Autodesk Inventor part; units mm, degrees
(part 2 of 2)
  spline S10 degree 5 poles (30.7335, -5.459) (30.6894, -5.4223) (30.6454, -5.3856) (30.6013, -5.349) (30.5128, -5.276) (30.4236, -5.2038) (30.3788, -5.168) (30.2889, -5.0968) (30.198, -5.0268) (30.1524, -4.992) (30.0608, -4.9229) (29.9686, -4.8547) (29.9224, -4.8208) (29.8295, -4.7535) (29.7359, -4.6872) (29.6889, -4.6543) (29.5946, -4.589) (29.4996, -4.5247) (29.4519, -4.4929) (29.3561, -4.4297) (29.2597, -4.3677) (29.2112, -4.3369) (29.114, -4.2761) (29.016, -4.2164) (28.9669, -4.1869) (28.8682, -4.1285) (28.7687, -4.0713) (28.7188, -4.0431) (28.6186, -3.9873) (28.5176, -3.9329) (28.4669, -3.906) (28.3651, -3.8531) (28.2626, -3.8017) (28.2111, -3.7764) (28.1077, -3.7267) (28.0035, -3.6787) (27.9512, -3.6551) (27.8462, -3.6092) (27.7402, -3.5651) (27.6871, -3.5436) (27.5804, -3.5014) (27.4729, -3.4613) (27.419, -3.4418) (27.3105, -3.4043) (27.201, -3.3704) (27.1459, -3.3543) (27.0348, -3.3257) (26.9231, -3.2995) (26.8672, -3.2864) (26.7557, -3.2591) (26.6453, -3.2277) (26.5905, -3.2106) (26.4821, -3.1729) (26.3763, -3.1281) (26.3244, -3.1036) (26.2219, -3.0515) (26.1238, -2.9918) (26.0756, -2.9603) (25.983, -2.8924) (25.8981, -2.8146) (25.8596, -2.7722) (25.7804, -2.6886) (25.7171, -2.5923) (25.6878, -2.5432) (25.6326, -2.442) (25.5979, -2.3325) (25.5767, -2.2787) (25.5598, -2.1649) (25.5445, -2.0515) (25.5485, -1.9934) (25.5547, -1.8796) (25.5649, -1.7651) (25.5676, -1.7081) (25.5752, -1.5936) (25.5834, -1.4798) (25.5913, -1.4224) (25.6225, -1.3127) (25.658, -1.2036) (25.6879, -1.1544) (25.737, -1.0509) (25.8098, -0.9618) (25.8435, -0.916) (25.9234, -0.8334) (26.0119, -0.7613) (26.0571, -0.7261) (26.1519, -0.6617) (26.2538, -0.6093) (26.3056, -0.5851) (26.411, -0.5405) (26.5196, -0.5041) (26.5744, -0.4877) (26.6851, -0.4586) (26.7974, -0.4368) (26.8539, -0.4278) (26.9673, -0.4125) (27.0811, -0.4011) (27.138, -0.3958) (27.2519, -0.385) (27.3654, -0.3711) (27.4219, -0.3624) (27.5347, -0.3434) (27.6467, -0.3208) (27.7026, -0.3088) (27.8141, -0.2835) (27.9251, -0.2561) (27.9804, -0.2419) (28.0909, -0.2126) (28.2008, -0.1814) (28.2556, -0.1651) (28.3649, -0.1317) (28.4736, -0.0965) (28.5278, -0.0785) (28.6359, -0.0416) (28.7435, -0.003) (28.7971, 0.0167) (28.9041, 0.0568) (29.0106, 0.0983) (29.0637, 0.1195) (29.1695, 0.1625) (29.2748, 0.2068) (29.3274, 0.2293) (29.4321, 0.275) (29.5363, 0.3219) (29.5882, 0.3457) (29.6918, 0.3939) (29.7949, 0.4433) (29.8462, 0.4683) (29.9487, 0.5189) (30.0506, 0.5706) (30.1014, 0.5967) (30.2028, 0.6495) (30.3036, 0.7033) (30.3538, 0.7305) (30.4541, 0.7854) (30.5538, 0.8412) (30.6035, 0.8693) (30.7026, 0.9261) (30.8011, 0.9841) (30.8501, 1.0134) (30.9479, 1.0726) (31.0451, 1.1326) (31.0937, 1.1628) (31.1421, 1.193) (31.1906, 1.2233) knots 0 0 0 0 0 0 0.021315 0.021315 0.021315 0.04263 0.04263 0.04263 0.063945 0.063945 0.063945 0.08526 0.08526 0.08526 0.106575 0.106575 0.106575 0.12789 0.12789 0.12789 0.149204 0.149204 0.149204 0.170519 0.170519 0.170519 0.191835 0.191835 0.191835 0.21315 0.21315 0.21315 0.234465 0.234465 0.234465 0.255779 0.255779 0.255779 0.277094 0.277094 0.277094 0.298412 0.298412 0.298412 0.319724 0.319724 0.319724 0.341052 0.341052 0.341052 0.362374 0.362374 0.362374 0.383705 0.383705 0.383705 0.405045 0.405045 0.405045 0.42637 0.42637 0.42637 0.447676 0.447676 0.447676 0.468973 0.468973 0.468973 0.490261 0.490261 0.490261 0.511544 0.511544 0.511544 0.532795 0.532795 0.532795 0.554 0.554 0.554 0.575212 0.575212 0.575212 0.596458 0.596458 0.596458 0.617711 0.617711 0.617711 0.63897 0.63897 0.63897 0.660221 0.660221 0.660221 0.681474 0.681474 0.681474 0.702716 0.702716 0.702716 0.723962 0.723962 0.723962 0.745198 0.745198 0.745198 0.76643 0.76643 0.76643 0.787663 0.787663 0.787663 0.808897 0.808897 0.808897 0.830131 0.830131 0.830131 0.851365 0.851365 0.851365 0.872598 0.872598 0.872598 0.893831 0.893831 0.893831 0.915065 0.915065 0.915065 0.936299 0.936299 0.936299 0.957533 0.957533 0.957533 0.978766 0.978766 0.978766 1 1 1 1 1 1 projected
  arc A22 (31.1906, 1.2233) -> (31.0667, 3.0352) centre (0, 0) ccw projected
  spline S11 degree 5 poles (31.0667, 3.0352) (31.0143, 3.0587) (30.962, 3.0821) (30.9096, 3.1055) (30.8047, 3.1519) (30.6994, 3.1974) (30.6466, 3.2198) (30.5408, 3.264) (30.4344, 3.307) (30.3811, 3.3281) (30.2743, 3.3699) (30.1671, 3.4108) (30.1134, 3.4309) (30.0058, 3.4707) (29.8978, 3.5093) (29.8437, 3.5283) (29.7352, 3.5657) (29.6264, 3.6019) (29.5719, 3.6198) (29.4627, 3.6547) (29.353, 3.6885) (29.2981, 3.705) (29.1881, 3.7374) (29.0776, 3.7684) (29.0223, 3.7835) (28.9115, 3.8132) (28.8003, 3.8414) (28.7446, 3.8551) (28.6331, 3.8818) (28.5211, 3.9069) (28.4651, 3.9191) (28.3528, 3.9426) (28.2402, 3.9644) (28.1838, 3.9749) (28.0709, 3.9949) (27.9576, 4.013) (27.9009, 4.0216) (27.7873, 4.0375) (27.6734, 4.0513) (27.6164, 4.0577) (27.5023, 4.0696) (27.388, 4.0792) (27.3308, 4.0833) (27.2163, 4.0902) (27.1016, 4.0933) (27.0442, 4.094) (26.9295, 4.0915) (26.8149, 4.0866) (26.7576, 4.0841) (26.6428, 4.0804) (26.5281, 4.0808) (26.4707, 4.0825) (26.3561, 4.0895) (26.2421, 4.1041) (26.1856, 4.1137) (26.0728, 4.1362) (25.9623, 4.1673) (25.9073, 4.1846) (25.7999, 4.225) (25.6971, 4.277) (25.6485, 4.3075) (25.5498, 4.3666) (25.4629, 4.4422) (25.4214, 4.4816) (25.3409, 4.5642) (25.278, 4.6602) (25.243, 4.7063) (25.1961, 4.8113) (25.1508, 4.9164) (25.1389, 4.9734) (25.1142, 5.0847) (25.0931, 5.1977) (25.0804, 5.2533) (25.0567, 5.3655) (25.0339, 5.4774) (25.0261, 5.5348) (25.0265, 5.6488) (25.0312, 5.7634) (25.0468, 5.8189) (25.0661, 5.9318) (25.1122, 6.0373) (25.1323, 6.0905) (25.1869, 6.1915) (25.2527, 6.2848) (25.2868, 6.3309) (25.3606, 6.4185) (25.4446, 6.4965) (25.488, 6.5338) (25.5775, 6.6051) (25.6721, 6.6695) (25.7205, 6.7001) (25.8192, 6.758) (25.9216, 6.8092) (25.9735, 6.8332) (26.0786, 6.8785) (26.1851, 6.9202) (26.2385, 6.9406) (26.3452, 6.9818) (26.4507, 7.0257) (26.5028, 7.0493) (26.6062, 7.0981) (26.7081, 7.1501) (26.7586, 7.1768) (26.8592, 7.2311) (26.9586, 7.2875) (27.0081, 7.3161) (27.1066, 7.3741) (27.204, 7.4338) (27.2523, 7.4643) (27.3486, 7.5259) (27.4437, 7.5891) (27.4911, 7.6211) (27.5852, 7.6858) (27.6784, 7.752) (27.7248, 7.7854) (27.817, 7.8529) (27.9083, 7.9216) (27.9537, 7.9563) (28.044, 8.0263) (28.1335, 8.0974) (28.1779, 8.1332) (28.2665, 8.2055) (28.3541, 8.2788) (28.3977, 8.3157) (28.4845, 8.3901) (28.5704, 8.4655) (28.6131, 8.5034) (28.6981, 8.5797) (28.7823, 8.657) (28.8242, 8.6959) (28.9075, 8.774) (28.9901, 8.8531) (29.0311, 8.8928) (29.1128, 8.9727) (29.1938, 9.0533) (29.2341, 9.0938) (29.3142, 9.1753) (29.3934, 9.2577) (29.4327, 9.2991) (29.5109, 9.3825) (29.5883, 9.4665) (29.6269, 9.5086) (29.6654, 9.5508) (29.7039, 9.593) knots 0 0 0 0 0 0 0.021315 0.021315 0.021315 0.04263 0.04263 0.04263 0.063945 0.063945 0.063945 0.08526 0.08526 0.08526 0.106575 0.106575 0.106575 0.12789 0.12789 0.12789 0.149204 0.149204 0.149204 0.170519 0.170519 0.170519 0.191835 0.191835 0.191835 0.21315 0.21315 0.21315 0.234465 0.234465 0.234465 0.255779 0.255779 0.255779 0.277094 0.277094 0.277094 0.298412 0.298412 0.298412 0.319724 0.319724 0.319724 0.341052 0.341052 0.341052 0.362374 0.362374 0.362374 0.383705 0.383705 0.383705 0.405045 0.405045 0.405045 0.42637 0.42637 0.42637 0.447676 0.447676 0.447676 0.468973 0.468973 0.468973 0.490261 0.490261 0.490261 0.511544 0.511544 0.511544 0.532795 0.532795 0.532795 0.554 0.554 0.554 0.575212 0.575212 0.575212 0.596458 0.596458 0.596458 0.617711 0.617711 0.617711 0.63897 0.63897 0.63897 0.660221 0.660221 0.660221 0.681474 0.681474 0.681474 0.702716 0.702716 0.702716 0.723962 0.723962 0.723962 0.745198 0.745198 0.745198 0.76643 0.76643 0.76643 0.787663 0.787663 0.787663 0.808897 0.808897 0.808897 0.830131 0.830131 0.830131 0.851365 0.851365 0.851365 0.872598 0.872598 0.872598 0.893831 0.893831 0.893831 0.915065 0.915065 0.915065 0.936299 0.936299 0.936299 0.957533 0.957533 0.957533 0.978766 0.978766 0.978766 1 1 1 1 1 1 projected
  arc A23 (29.7039, 9.593) -> (29.0957, 11.3044) centre (0, 0) ccw projected
  spline S12 degree 5 poles (29.0957, 11.3044) (29.039, 11.3128) (28.9823, 11.3213) (28.9255, 11.3297) (28.812, 11.346) (28.6983, 11.3614) (28.6415, 11.3688) (28.5276, 11.3828) (28.4136, 11.3955) (28.3566, 11.4014) (28.2424, 11.4129) (28.1282, 11.4233) (28.0711, 11.4282) (27.9567, 11.4374) (27.8423, 11.4454) (27.7851, 11.4492) (27.6706, 11.456) (27.556, 11.4615) (27.4987, 11.4639) (27.3841, 11.4682) (27.2694, 11.471) (27.2121, 11.4721) (27.0974, 11.4736) (26.9827, 11.4737) (26.9253, 11.4734) (26.8106, 11.472) (26.6959, 11.4691) (26.6386, 11.4673) (26.524, 11.4629) (26.4094, 11.457) (26.3522, 11.4536) (26.2377, 11.4459) (26.1234, 11.4365) (26.0663, 11.4314) (25.9521, 11.4202) (25.8382, 11.407) (25.7812, 11.4) (25.6676, 11.3847) (25.5542, 11.3673) (25.4976, 11.3581) (25.3845, 11.3387) (25.2718, 11.3171) (25.2156, 11.3057) (25.1035, 11.2814) (24.9922, 11.2534) (24.9368, 11.2386) (24.827, 11.2053) (24.718, 11.1696) (24.6634, 11.1518) (24.554, 11.1172) (24.4434, 11.0867) (24.3876, 11.0728) (24.2754, 11.0486) (24.1617, 11.032) (24.1047, 11.0259) (23.99, 11.0172) (23.8752, 11.0173) (23.8176, 11.0191) (23.7033, 11.0291) (23.5902, 11.0514) (23.5353, 11.0676) (23.4243, 11.0979) (23.3202, 11.1473) (23.2696, 11.174) (23.1698, 11.2318) (23.0833, 11.3073) (23.0372, 11.3423) (22.9637, 11.4307) (22.8917, 11.5197) (22.8649, 11.5713) (22.811, 11.6719) (22.7602, 11.775) (22.733, 11.8251) (22.6799, 11.9268) (22.6278, 12.0284) (22.6048, 12.0815) (22.5745, 12.1914) (22.548, 12.3031) (22.5481, 12.3606) (22.5362, 12.4746) (22.5521, 12.5886) (22.5572, 12.6452) (22.5825, 12.7573) (22.6206, 12.8649) (22.641, 12.9185) (22.6885, 13.0227) (22.7483, 13.1204) (22.78, 13.1681) (22.847, 13.2609) (22.9207, 13.3484) (22.9591, 13.3909) (23.0385, 13.4733) (23.1232, 13.5503) (23.1668, 13.5874) (23.2557, 13.6593) (23.347, 13.7282) (23.3929, 13.7623) (23.4846, 13.8307) (23.5744, 13.9015) (23.6181, 13.9383) (23.7046, 14.0131) (23.7886, 14.0907) (23.8301, 14.13) (23.9122, 14.2095) (23.9928, 14.2906) (24.0327, 14.3315) (24.1119, 14.4139) (24.1896, 14.4977) (24.2279, 14.5401) (24.3039, 14.6254) (24.3785, 14.7119) (24.4155, 14.7555) (24.4887, 14.8432) (24.5606, 14.9321) (24.5962, 14.9768) (24.6668, 15.0666) (24.7361, 15.1575) (24.7705, 15.2031) (24.8386, 15.2948) (24.9055, 15.3874) (24.9387, 15.434) (25.0045, 15.5274) (25.0691, 15.6216) (25.1011, 15.669) (25.1646, 15.764) (25.227, 15.8597) (25.2579, 15.9078) (25.3191, 16.0042) (25.3793, 16.1013) (25.4092, 16.1501) (25.4684, 16.2478) (25.5265, 16.3462) (25.5553, 16.3955) (25.6125, 16.4945) (25.6687, 16.594) (25.6966, 16.6438) (25.7517, 16.7439) (25.8057, 16.8446) (25.8324, 16.8951) (25.8852, 16.9965) (25.9371, 17.0983) (25.9629, 17.1493) (25.9886, 17.2003) (26.0143, 17.2513) knots 0 0 0 0 0 0 0.021315 0.021315 0.021315 0.04263 0.04263 0.04263 0.063945 0.063945 0.063945 0.08526 0.08526 0.08526 0.106575 0.106575 0.106575 0.12789 0.12789 0.12789 0.149204 0.149204 0.149204 0.170519 0.170519 0.170519 0.191835 0.191835 0.191835 0.21315 0.21315 0.21315 0.234465 0.234465 0.234465 0.255779 0.255779 0.255779 0.277094 0.277094 0.277094 0.298412 0.298412 0.298412 0.319724 0.319724 0.319724 0.341052 0.341052 0.341052 0.362374 0.362374 0.362374 0.383705 0.383705 0.383705 0.405045 0.405045 0.405045 0.42637 0.42637 0.42637 0.447676 0.447676 0.447676 0.468973 0.468973 0.468973 0.490261 0.490261 0.490261 0.511544 0.511544 0.511544 0.532795 0.532795 0.532795 0.554 0.554 0.554 0.575212 0.575212 0.575212 0.596458 0.596458 0.596458 0.617711 0.617711 0.617711 0.63897 0.63897 0.63897 0.660221 0.660221 0.660221 0.681474 0.681474 0.681474 0.702716 0.702716 0.702716 0.723962 0.723962 0.723962 0.745198 0.745198 0.745198 0.76643 0.76643 0.76643 0.787663 0.787663 0.787663 0.808897 0.808897 0.808897 0.830131 0.830131 0.830131 0.851365 0.851365 0.851365 0.872598 0.872598 0.872598 0.893831 0.893831 0.893831 0.915065 0.915065 0.915065 0.936299 0.936299 0.936299 0.957533 0.957533 0.957533 0.978766 0.978766 0.978766 1 1 1 1 1 1 projected
  arc A24 (26.0143, 17.2513) -> (24.9669, 18.7351) centre (0, 0) ccw projected
  spline S13 degree 5 poles (24.9669, 18.7351) (24.91, 18.7279) (24.8531, 18.7208) (24.7962, 18.7136) (24.6825, 18.6987) (24.5689, 18.6828) (24.5121, 18.6745) (24.3987, 18.6573) (24.2855, 18.6388) (24.229, 18.6291) (24.116, 18.6094) (24.0032, 18.5886) (23.9468, 18.5779) (23.8342, 18.5559) (23.7219, 18.5328) (23.6658, 18.5209) (23.5537, 18.4966) (23.4419, 18.471) (23.386, 18.4579) (23.2745, 18.431) (23.1633, 18.4028) (23.1078, 18.3884) (22.997, 18.3589) (22.8865, 18.328) (22.8314, 18.3123) (22.7213, 18.28) (22.6116, 18.2463) (22.5569, 18.2291) (22.4477, 18.194) (22.339, 18.1573) (22.2848, 18.1386) (22.1767, 18.1003) (22.0691, 18.0605) (22.0155, 18.0401) (21.9086, 17.9985) (21.8024, 17.9551) (21.7495, 17.9329) (21.6442, 17.8875) (21.5397, 17.8402) (21.4877, 17.8161) (21.384, 17.7669) (21.2814, 17.7157) (21.2303, 17.6895) (21.1289, 17.6359) (21.0293, 17.579) (20.98, 17.5497) (20.8832, 17.488) (20.7878, 17.4243) (20.7401, 17.3923) (20.644, 17.3295) (20.5458, 17.2703) (20.4959, 17.2419) (20.3943, 17.1883) (20.2894, 17.1417) (20.236, 17.1204) (20.128, 17.0811) (20.0174, 17.0502) (19.9615, 17.0364) (19.8487, 17.0151) (19.7338, 17.0061) (19.6765, 17.0069) (19.5614, 17.0062) (19.4479, 17.0256) (19.392, 17.0377) (19.2803, 17.0665) (19.1766, 17.1158) (19.1228, 17.137) (19.0281, 17.2023) (18.9348, 17.2686) (18.8951, 17.3111) (18.8161, 17.3934) (18.7394, 17.479) (18.6996, 17.5199) (18.6211, 17.6035) (18.5435, 17.6872) (18.507, 17.7322) (18.4481, 17.8298) (18.3926, 17.9302) (18.3771, 17.9857) (18.3349, 18.0922) (18.3195, 18.2062) (18.309, 18.2622) (18.3032, 18.3769) (18.3109, 18.4908) (18.3161, 18.5479) (18.3336, 18.6611) (18.3649, 18.7713) (18.3826, 18.8257) (18.422, 18.9332) (18.4694, 19.0374) (18.4949, 19.0887) (18.5491, 19.1894) (18.6099, 19.2864) (18.6419, 19.3338) (18.7081, 19.4271) (18.7774, 19.5181) (18.8124, 19.5633) (18.8822, 19.6539) (18.9496, 19.7463) (18.9818, 19.7935) (19.0448, 19.8889) (19.1048, 19.9863) (19.1342, 20.0353) (19.1918, 20.134) (19.2475, 20.2338) (19.275, 20.284) (19.3289, 20.3847) (19.3811, 20.4864) (19.4066, 20.5375) (19.4568, 20.6401) (19.5053, 20.7436) (19.5291, 20.7956) (19.5759, 20.8998) (19.6212, 21.0047) (19.6434, 21.0574) (19.6871, 21.1629) (19.7294, 21.2691) (19.7502, 21.3223) (19.791, 21.429) (19.8305, 21.5363) (19.8499, 21.59) (19.888, 21.6977) (19.9248, 21.8059) (19.9429, 21.8601) (19.9783, 21.9687) (20.0126, 22.0778) (20.0294, 22.1324) (20.0623, 22.2418) (20.0941, 22.3515) (20.1097, 22.4065) (20.1403, 22.5166) (20.1698, 22.627) (20.1842, 22.6823) (20.2125, 22.793) (20.2398, 22.9039) (20.2532, 22.9595) (20.2793, 23.0707) (20.3041, 23.1823) (20.3162, 23.2381) (20.3397, 23.3499) (20.3622, 23.462) (20.3733, 23.518) (20.3842, 23.5741) (20.3952, 23.6302) knots 0 0 0 0 0 0 0.021315 0.021315 0.021315 0.04263 0.04263 0.04263 0.063945 0.063945 0.063945 0.08526 0.08526 0.08526 0.106575 0.106575 0.106575 0.12789 0.12789 0.12789 0.149204 0.149204 0.149204 0.170519 0.170519 0.170519 0.191835 0.191835 0.191835 0.21315 0.21315 0.21315 0.234465 0.234465 0.234465 0.255779 0.255779 0.255779 0.277094 0.277094 0.277094 0.298412 0.298412 0.298412 0.319724 0.319724 0.319724 0.341052 0.341052 0.341052 0.362374 0.362374 0.362374 0.383705 0.383705 0.383705 0.405045 0.405045 0.405045 0.42637 0.42637 0.42637 0.447676 0.447676 0.447676 0.468973 0.468973 0.468973 0.490261 0.490261 0.490261 0.511544 0.511544 0.511544 0.532795 0.532795 0.532795 0.554 0.554 0.554 0.575212 0.575212 0.575212 0.596458 0.596458 0.596458 0.617711 0.617711 0.617711 0.63897 0.63897 0.63897 0.660221 0.660221 0.660221 0.681474 0.681474 0.681474 0.702716 0.702716 0.702716 0.723962 0.723962 0.723962 0.745198 0.745198 0.745198 0.76643 0.76643 0.76643 0.787663 0.787663 0.787663 0.808897 0.808897 0.808897 0.830131 0.830131 0.830131 0.851365 0.851365 0.851365 0.872598 0.872598 0.872598 0.893831 0.893831 0.893831 0.915065 0.915065 0.915065 0.936299 0.936299 0.936299 0.957533 0.957533 0.957533 0.978766 0.978766 0.978766 1 1 1 1 1 1 projected
  arc A25 (20.3952, 23.6302) -> (18.9864, 24.7764) centre (0, 0) ccw projected
  spline S14 degree 5 poles (18.9864, 24.7764) (18.9335, 24.7541) (18.8807, 24.7319) (18.8278, 24.7095) (18.7223, 24.6645) (18.6172, 24.6186) (18.5648, 24.5953) (18.4602, 24.5481) (18.3562, 24.4998) (18.3044, 24.4752) (18.2009, 24.4257) (18.0979, 24.3752) (18.0466, 24.3497) (17.9441, 24.2982) (17.8421, 24.2456) (17.7913, 24.2191) (17.6899, 24.1654) (17.5892, 24.1106) (17.5389, 24.0829) (17.4388, 24.0269) (17.3393, 23.9698) (17.2898, 23.9409) (17.191, 23.8826) (17.093, 23.8231) (17.0441, 23.793) (16.9468, 23.7322) (16.8503, 23.6702) (16.8023, 23.6389) (16.7066, 23.5756) (16.6119, 23.511) (16.5647, 23.4783) (16.4709, 23.4123) (16.3781, 23.3449) (16.332, 23.3108) (16.2402, 23.2419) (16.1497, 23.1715) (16.1047, 23.1359) (16.0156, 23.0637) (15.9277, 22.99) (15.8841, 22.9527) (15.7976, 22.8774) (15.7125, 22.8004) (15.6705, 22.7614) (15.5873, 22.6824) (15.5067, 22.6007) (15.4671, 22.5592) (15.3906, 22.4737) (15.3159, 22.3866) (15.2786, 22.343) (15.2031, 22.2566) (15.1244, 22.173) (15.084, 22.1322) (15.0007, 22.0533) (14.9122, 21.98) (14.8666, 21.9452) (14.7732, 21.8782) (14.675, 21.8185) (14.6249, 21.7902) (14.522, 21.7393) (14.4138, 21.6996) (14.3584, 21.6849) (14.2478, 21.6531) (14.1333, 21.6412) (14.0762, 21.6378) (13.9609, 21.6354) (13.8477, 21.6549) (13.7902, 21.6608) (13.6814, 21.6982) (13.5736, 21.7368) (13.5239, 21.767) (13.4257, 21.8249) (13.3287, 21.8867) (13.2794, 21.9153) (13.1812, 21.9746) (13.0839, 22.0343) (13.0366, 22.0677) (12.9536, 22.1459) (12.873, 22.2276) (12.8431, 22.2768) (12.7738, 22.368) (12.7281, 22.4736) (12.703, 22.5247) (12.6664, 22.6336) (12.6431, 22.7453) (12.6327, 22.8017) (12.6191, 22.9154) (12.6195, 23.03) (12.6218, 23.0872) (12.6307, 23.2013) (12.6483, 23.3144) (12.659, 23.3706) (12.684, 23.4823) (12.7164, 23.5921) (12.7344, 23.6464) (12.773, 23.7541) (12.8152, 23.8604) (12.8367, 23.9134) (12.8794, 24.0194) (12.9194, 24.1266) (12.9377, 24.1808) (12.9726, 24.2896) (13.0041, 24.3995) (13.0192, 24.4547) (13.048, 24.5653) (13.0748, 24.6764) (13.0876, 24.7321) (13.1124, 24.8437) (13.1352, 24.9556) (13.146, 25.0117) (13.1667, 25.1241) (13.1854, 25.2368) (13.1943, 25.2933) (13.2113, 25.4063) (13.2266, 25.5195) (13.2338, 25.5762) (13.2474, 25.6897) (13.2594, 25.8033) (13.2651, 25.8602) (13.2756, 25.9739) (13.2847, 26.0879) (13.2889, 26.1448) (13.2965, 26.2588) (13.3028, 26.3729) (13.3055, 26.43) (13.3104, 26.5442) (13.3139, 26.6584) (13.3154, 26.7155) (13.3176, 26.8297) (13.3186, 26.944) (13.3188, 27.0011) (13.3185, 27.1154) (13.3171, 27.2297) (13.3161, 27.2868) (13.3135, 27.401) (13.3099, 27.5152) (13.3078, 27.5723) (13.3029, 27.6865) (13.2967, 27.8006) (13.2932, 27.8576) (13.2857, 27.9717) (13.2772, 28.0856) (13.2727, 28.1426) (13.2681, 28.1995) (13.2636, 28.2565) knots 0 0 0 0 0 0 0.021315 0.021315 0.021315 0.04263 0.04263 0.04263 0.063945 0.063945 0.063945 0.08526 0.08526 0.08526 0.106575 0.106575 0.106575 0.12789 0.12789 0.12789 0.149204 0.149204 0.149204 0.170519 0.170519 0.170519 0.191835 0.191835 0.191835 0.21315 0.21315 0.21315 0.234465 0.234465 0.234465 0.255779 0.255779 0.255779 0.277094 0.277094 0.277094 0.298412 0.298412 0.298412 0.319724 0.319724 0.319724 0.341052 0.341052 0.341052 0.362374 0.362374 0.362374 0.383705 0.383705 0.383705 0.405045 0.405045 0.405045 0.42637 0.42637 0.42637 0.447676 0.447676 0.447676 0.468973 0.468973 0.468973 0.490261 0.490261 0.490261 0.511544 0.511544 0.511544 0.532795 0.532795 0.532795 0.554 0.554 0.554 0.575212 0.575212 0.575212 0.596458 0.596458 0.596458 0.617711 0.617711 0.617711 0.63897 0.63897 0.63897 0.660221 0.660221 0.660221 0.681474 0.681474 0.681474 0.702716 0.702716 0.702716 0.723962 0.723962 0.723962 0.745198 0.745198 0.745198 0.76643 0.76643 0.76643 0.787663 0.787663 0.787663 0.808897 0.808897 0.808897 0.830131 0.830131 0.830131 0.851365 0.851365 0.851365 0.872598 0.872598 0.872598 0.893831 0.893831 0.893831 0.915065 0.915065 0.915065 0.936299 0.936299 0.936299 0.957533 0.957533 0.957533 0.978766 0.978766 0.978766 1 1 1 1 1 1 projected
  arc A26 (13.2636, 28.2565) -> (11.5977, 28.98) centre (0, 0) ccw projected
  line L2 (-24.5853, -10.152) -> (-4.701, 5.8438)
  line L3 (4.701, 5.8438) -> (24.5853, -10.152)
  arc A27 (4.701, 5.8438) -> (-4.701, 5.8438) centre (0, 0) ccw
  point P0 (20.9346, -16.4086)
  point P1 (6.1034, 4.3588)
  dimension "d19" = 120
  dimension "d20" = 15
  constraints: 8 end point, 5 point on circle, 2 centre point, 2 tangent, 1 coincident, 1 concentric, 1 horizontal alignment, 34 other
  measures "d19" angle of L1 L0
  measures "d20" diameter of A2
extrude "Extrusion5" cut sketch "Sketch4" against normal through all contours A26 S14 A25 S13 A24 S12 A23 S11 A22 S10 A21 S9 L3 A27 L2 S8 A11 S7 A10 S6 A9 S5 A8 S4 A7 S3 A6 S2 A5 S1 A4 S0
equation "\"d0\" = FaceWidth"
equation "\"Module\" = 2.5"
equation "\"PressureAngle\" = 20deg"
equation "\"UnitProfileClearance\" = 0.25"
equation "\"UnitRoundRadius\" = 0.35"
equation "\"HeadDiameter\" = 62.42917"
equation "\"RootDiameter\" = 51.25"
equation "\"BaseDiameter\" = 54.03233"
equation "\"PitchDiameter\" = 57.5"
equation "\"FaceWidth\" = 8"
equation "\"HelixAngle\" = 0"
equation "\"UnitCorrection\" = 0"
equation "\"UnitAddendumModification\" = 0.014165"
equation "\"CircularPitch\" = 7.853982"
equation "\"UnitBacklashShift\" = 0"
equation "\"TotalToolShift\" = 0"
equation "\"IsInternal\" = 0"
body "Solid1"
